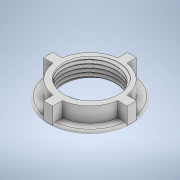
# Autodesk Inventor part: Connector Female
Saved by Autodesk Inventor 2020.2 (Build 242310000, 310)
## iProperties
Created: 2020-04-22
Part Number: Connector Female
Material: Generic
Document SubType Name: Modeling
Designer: a
Density: 1 g/cm^3
Appearance: Default
Author: a
Autodesk Inventor part; units mm, degrees
ref_plane "YZ Plane" through (0, 0, 0) normal (1, 0, 0) x (0, 1, 0)
ref_plane "XZ Plane" through (0, 0, 0) normal (0, 1, 0) x (-1, 0, 0)
ref_plane "XY Plane" through (0, 0, 0) normal (0, 0, 1) x (1, 0, 0)
sketch "Sketch1" plane through (0, 0, 0) normal (0, 1, 0) x (-1, 0, 0)
  circle A0 centre (0, 0) radius 22.5
  circle A1 centre (0, 0) radius 14.0171
  dimension "d0" = 45
  dimension "d1" = 28.0342
  constraints: 2 centre point, 2 coincident
  measures "d0" diameter of A0
  measures "d1" diameter of A1
extrude "Extrusion1" add sketch "Sketch1" along normal blind 2
sketch "Sketch2" plane through (0, 2, 0) normal (0, 1, 0) x (1, 0, 0)
  circle A0 centre (0, 0) radius 17.5
  circle A1 centre (0, 0) radius 14.0171
  circle A2 centre (0, 0) radius 14.0171 projected
  line L0 (-17.3205, -2.5) -> (-22.3607, -2.5)
  circle A3 centre (0, 0) radius 22.5 projected
  line L1 (-17.3205, 2.5) -> (-22.3607, 2.5)
  arc A4 (-22.3607, 2.5) -> (-22.3607, -2.5) centre (0, 0) ccw
  line L2 (-31.5, 0) -> (31.5, 0) projected
  line L3 (-2.5, -17.3205) -> (-2.5, -22.3607)
  arc A5 (-2.5, -22.3607) -> (2.5, -22.3607) centre (0, 0) ccw
  line L4 (2.5, -17.3205) -> (2.5, -22.3607)
  line L5 (17.3205, -2.5) -> (22.3607, -2.5)
  arc A6 (22.3607, -2.5) -> (22.3607, 2.5) centre (0, 0) ccw
  line L6 (17.3205, 2.5) -> (22.3607, 2.5)
  line L7 (2.5, 17.3205) -> (2.5, 22.3607)
  arc A7 (2.5, 22.3607) -> (-2.5, 22.3607) centre (0, 0) ccw
  line L8 (-2.5, 17.3205) -> (-2.5, 22.3607)
  dimension "d4" = 35
  dimension "d9" = 5
  dimension "d12" = 360
  constraints: 16 end point, 12 point on circle, 6 centre point, 2 coincident, 2 concentric, 1 horizontal, 1 parallel, 34 other
  measures "d4" diameter of A0
  measures "d9" distance between parallel lines of L1 L0
extrude "Extrusion2" add sketch "Sketch2" along normal blind 8 contours L2 A1 A0 | L2 A3 L5 A0 | A0 L2 A1 | A0 L6 A3 L2 | A0 L8 A3 L7 | L4 A3 L3 A0 | L2 A3 L1 A0 | A0 L0 A3 L2
fillet "Fillet1" radius 1 5 edges at (15.9099, 2, 15.9099) (-15.9099, 2, 15.9099) (-15.9099, 2, -15.9099) (15.9099, 2, -15.9099) (22.5, 0, 0)
thread "Thread7" size "M30x2" class "6H" standard "ANSI Metric M Profile" full length
sketch "Sketch13" plane through (0, 10, 15.15) normal (-1, 0, 0) x (0, -1, 0)
  line L0 (-1.1668, 0.2486) -> (-1.0001, 0.2486) construction
  line L1 (0.1666, -1.0321) -> (-0.0001, -1.3523) construction
  line L2 (-2.0001, -1.3523) -> (-2.1668, -1.0321) construction
  line L3 (-0.8334, 0.2486) -> (-1.0001, 0.5687) construction
  line L4 (-1.0001, 0.5687) -> (-1.1668, 0.2486) construction
  line L5 (-2.0001, -1.3523) -> (-1.8334, -1.0321) construction
  line L6 (-0.8334, 0.2486) -> (-0.1668, -1.0321)
  line L7 (-2.1668, -1.0321) -> (-1.8334, -1.0321) construction
  arc A0 (-2.1668, -1.0321) -> (-2.0001, -1.1332) centre (-2.0001, -0.9453) ccw construction
  line L8 (0.1666, -1.0321) -> (-0.1668, -1.0321) construction
  line L9 (-2.0001, -1.3523) -> (-2.0001, -1.0321) construction
  line L10 (-0.0001, -1.3523) -> (-0.0001, -1.0321) construction
  line L11 (-1.0001, 0.5687) -> (-1.0001, 0.3497) construction
  line L12 (-2.0001, -1.1332) -> (-0.0001, -1.1332)
  arc A1 (-2.0001, -1.1332) -> (-1.8334, -1.0321) centre (-2.0001, -0.9453) ccw
  line L13 (-0.1668, -1.0321) -> (-0.0001, -1.3523) construction
  line L14 (-1.8334, -1.0321) -> (-1.1668, 0.2486)
  line L15 (-0.0001, 0.3497) -> (-0.0001, 0.3675)
  line L16 (-0.0001, 0.3675) -> (-0.0001, 0.3497)
  line L17 (-0.0001, 0.3497) -> (0.0334, 0.3497)
  arc A2 (-0.1668, -1.0321) -> (-0.0001, -1.1332) centre (-0.0001, -0.9453) ccw
  arc A3 (-0.0001, -1.1332) -> (0.1666, -1.0321) centre (-0.0001, -0.9453) ccw construction
  arc A4 (-1.0001, 0.3497) -> (-1.1668, 0.2486) centre (-1.0001, 0.1618) ccw
  arc A5 (-0.8334, 0.2486) -> (-1.0001, 0.3497) centre (-1.0001, 0.1618) ccw
  line L18 (-1.0001, 0.3497) -> (-1.0001, 0.2486) construction
  line L19 (-1.0001, 0.2486) -> (-0.8334, 0.2486) construction
  dimension "d118" = 55
  dimension "d119" = 0.3202
  dimension "d120" = 0.3202
  dimension "Sketch13_ThreadOffset" = 0
  dimension "Sketch13_MajorRadius" = 1.4829
  dimension "d123" = 2
  dimension "Sketch13_MinorRadius" = 0
  constraints: 40 end point, 12 point on circle, 10 parallel, 8 tangent, 6 centre point, 6 collinear, 2 midpoint, 2 point on line, 1 horizontal, 1 perpendicular
  measures "d118" angle of L6 L14
  measures "d119" distance of L3.end L0.end
  measures "d120" distance of L1.end L10.end
  measures "Sketch13_ThreadOffset" distance between parallel lines of L15 L10
  measures "Sketch13_MajorRadius" distance from line of L12 L15.start
  measures "d123" distance from line of L1.end L9
  measures "Sketch13_MinorRadius" distance edge to line of A5 L17
sketch "Sketch14" plane through (0, 10, 0) normal (1, 0, 0) x (0, 0, 1)
  line L0 (15.15, 0) -> (15.15, 10)
  line L1 (15.15, 10) -> (13.6671, 10)
  line L2 (13.6671, 10) -> (13.6671, 0)
  line L3 (13.6671, 0) -> (15.15, 0)
  line L4 (0, -2) -> (0, 12) projected
  constraints: 8 end point
revolve "Revolution6" [suppressed]
coil "Coil6" sketch "Sketch13" operation cut axis through (0, 10, 0) along (0, -1, 0) pitch 2.002 turns 6.993007 hand right
equation "\"d118\" = d125"
equation "\"d119\" = 0.160083 * Sketch13_Pitch"
equation "\"d120\" = 0.160083 * Sketch13_Pitch"
equation "\"d123\" = Sketch13_Pitch"
equation "\"d23\" = 55deg"
equation "\"Sketch3_Pitch\" = 1"
equation "\"d43\" = 55deg"
equation "\"Sketch5_Pitch\" = 1"
equation "\"d63\" = 55deg"
equation "\"Sketch7_Pitch\" = 1"
equation "\"d83\" = 55deg"
equation "\"Sketch9_Pitch\" = 1"
equation "\"d104\" = 55deg"
equation "\"Sketch11_Pitch\" = 2"
equation "\"d125\" = 55deg"
equation "\"Sketch13_Pitch\" = 2"
body "Solid1"
body "Solid7"
